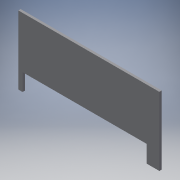
# Autodesk Inventor part: PCBWall
Saved by Autodesk Inventor 2017 (Build 210142000, 142)
## iProperties
Created: 2017-03-28
Part Number: PCBWall
Material: Generic
Document SubType Name: Modeling
Designer: hoeflinc
Density: 1 g/cm^3
Appearance: Default
Author: hoeflinc
Quantity: 1
Autodesk Inventor part; units mm, degrees
ref_plane "YZ Plane" through (0, 0, 0) normal (1, 0, 0) x (0, 1, 0)
ref_plane "XZ Plane" through (0, 0, 0) normal (0, 1, 0) x (-1, 0, 0)
ref_plane "XY Plane" through (0, 0, 0) normal (0, 0, 1) x (1, 0, 0)
sketch "Sketch1" plane through (0, 0, 0) normal (0, 0, 1) x (1, 0, 0)
  line L0 (0, 0) -> (209.2198, 0)
  line L1 (209.2198, 0) -> (209.2198, 101.6)
  line L2 (209.2198, 101.6) -> (0, 101.6)
  line L3 (0, 101.6) -> (0, 0)
  dimension "d0" = 209.2198
  dimension "d1" = 101.6
  constraints: 8 end point, 2 parallel, 1 horizontal, 1 perpendicular
  measures "d0" distance of L1.end L2.end
  measures "d1" distance of L2.end L0.start
extrude "Extrusion1" add sketch "Sketch1" along normal blind 3.5
sketch "Sketch2" plane through (0, 0, 3.5) normal (0, 0, 1) x (1, 0, 0)
  line L0 (6.35, 0) -> (190.5, 0)
  line L1 (190.5, 0) -> (190.5, 25.4)
  line L2 (190.5, 25.4) -> (6.35, 25.4)
  line L3 (6.35, 25.4) -> (6.35, 0)
  line L4 (0, 0) -> (209.2198, 0) projected
  line L5 (209.2198, 0) -> (209.2198, 101.6) projected
  line L6 (209.2198, 101.6) -> (0, 101.6) projected
  line L7 (0, 101.6) -> (0, 0) projected
  dimension "d4" = 25.4
  dimension "d5" = 184.15
  dimension "d6" = 6.35
  constraints: 8 end point, 2 parallel, 1 horizontal, 1 perpendicular
  measures "d4" distance of L2.end L0.start
  measures "d5" distance of L1.end L2.end
  measures "d6" distance between parallel lines of L7 L3
extrude "Extrusion2" cut sketch "Sketch2" against normal blind 3.5 contours L3 L2 L1 L0
body "Solid1"
